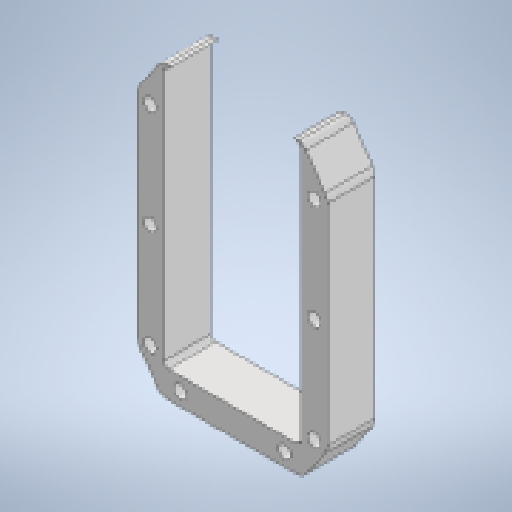
# Autodesk Inventor part: 부품70
Saved by Autodesk Inventor 2024 (Build 280153000, 153)
## iProperties
Created: 2024-09-08
Part Number: 부품70
Material: 일반
Document SubType Name: Modeling
Designer: Eungang
Density: 1 g/cm^3
Appearance: 기본값
Author: Eungang
Autodesk Inventor part; units mm, degrees
ref_plane "YZ Plane" through (0, 0, 0) normal (1, 0, 0) x (0, 1, 0)
ref_plane "XZ Plane" through (0, 0, 0) normal (0, 1, 0) x (-1, 0, 0)
ref_plane "XY Plane" through (0, 0, 0) normal (0, 0, 1) x (1, 0, 0)
sketch "스케치1" plane through (0, 0, 0) normal (0, 0, 1) x (1, 0, 0)
  arc A0 (19.8825, 4.0579) -> (19.3633, 5.7448) centre (16.8825, 4.0579) ccw projected
  line L0 (19.3633, 5.7448) -> (15.3778, 11.6059) projected
  arc A1 (15.3778, 11.6059) -> (13.7239, 12.4812) centre (13.7239, 10.4812) ccw projected
  line L1 (12.7825, 12.4812) -> (13.7239, 12.4812) projected
  arc A2 (14.2825, 10.9812) -> (12.7825, 12.4812) centre (12.7825, 10.9812) ccw projected
  line L2 (14.2825, -42.0188) -> (14.2825, 10.9812) projected
  arc A3 (13.2825, -43.0188) -> (14.2825, -42.0188) centre (13.2825, -42.0188) ccw projected
  line L3 (-13.7175, -43.0188) -> (13.2825, -43.0188) projected
  arc A4 (-14.7175, -42.0188) -> (-13.7175, -43.0188) centre (-13.7175, -42.0188) ccw projected
  line L4 (-14.7175, 10.9812) -> (-14.7175, -42.0188) projected
  arc A5 (-13.2175, 12.4812) -> (-14.7175, 10.9812) centre (-13.2175, 10.9812) ccw projected
  line L5 (-14.1589, 12.4812) -> (-13.2175, 12.4812) projected
  arc A6 (-14.1589, 12.4812) -> (-15.8128, 11.6059) centre (-14.1589, 10.4812) ccw projected
  line L6 (-15.8128, 11.6059) -> (-19.7983, 5.7448) projected
  arc A7 (-19.7983, 5.7448) -> (-20.3175, 4.0579) centre (-17.3175, 4.0579) ccw projected
  line L7 (-20.3175, 4.0579) -> (-20.3175, -40.1954) projected
  arc A8 (-20.3175, -40.1954) -> (-19.7983, -41.8823) centre (-17.3175, -40.1954) ccw projected
  line L8 (-19.7983, -41.8823) -> (-16.1104, -47.3057) projected
  arc A9 (-16.1104, -47.3057) -> (-13.6296, -48.6188) centre (-13.6296, -45.6188) ccw projected
  line L9 (-13.6296, -48.6188) -> (13.1946, -48.6188) projected
  arc A10 (13.1946, -48.6188) -> (15.6754, -47.3057) centre (13.1946, -45.6188) ccw projected
  line L10 (15.6754, -47.3057) -> (19.3633, -41.8823) projected
  arc A11 (19.3633, -41.8823) -> (19.8825, -40.1954) centre (16.8825, -40.1954) ccw projected
  line L11 (19.8825, -40.1954) -> (19.8825, 4.0579) projected
  circle A12 centre (-17.5175, 3.4812) radius 1.35 projected
  circle A13 centre (-17.5175, -18.5188) radius 1.35 projected
  circle A14 centre (-11.2175, -45.8188) radius 1.35 projected
  circle A15 centre (17.0825, 3.4812) radius 1.35 projected
  circle A16 centre (17.0825, -18.5188) radius 1.35 projected
  circle A17 centre (10.7825, -45.8188) radius 1.35 projected
  circle A18 centre (-17.5175, -40.5188) radius 1.35 projected
  circle A19 centre (17.0825, -40.5188) radius 1.35 projected
  circle A20 centre (-0.2175, -0.5188) radius 13.9 projected
  line L12 (25.5233, 26.6812) -> (19.5233, 26.6812) projected
  line L13 (19.5233, 26.6812) -> (19.5233, -57.2188) projected
  line L14 (25.5233, -57.2188) -> (19.5233, -57.2188) projected
  line L15 (25.5233, 26.6812) -> (25.5233, -57.2188) projected
  line L16 (-20.5175, 26.6812) -> (-26.5175, 26.6812) projected
  line L17 (-26.5175, 26.6812) -> (-26.5175, -57.2188) projected
  line L18 (-20.5175, -57.2188) -> (-26.5175, -57.2188) projected
  line L19 (-20.5175, 26.6812) -> (-20.5175, -57.2188) projected
  line L20 (14.2825, -40.5188) -> (19.5233, -40.5188)
  line L21 (19.5233, -40.5188) -> (19.5233, -57.2188)
  line L22 (19.5233, -57.2188) -> (14.2825, -57.2188)
  line L23 (14.2825, -57.2188) -> (14.2825, -40.5188)
  line L24 (-20.3, -40.5188) -> (-14.7175, -40.5188)
  line L25 (-14.7175, -40.5188) -> (-14.7175, -57.2188)
  line L26 (-14.7175, -57.2188) -> (-20.3, -57.2188)
  line L27 (-20.3, -57.2188) -> (-20.3, -40.5188)
  line L28 (19.865, -40.5188) -> (14.2825, -40.5188)
  line L29 (14.2825, -40.5188) -> (14.2825, -57.2188)
  line L30 (14.2825, -57.2188) -> (19.865, -57.2188)
  line L31 (19.865, -57.2188) -> (19.865, -40.5188)
  line L32 (-20.5175, -40.5188) -> (-14.7175, -40.5188)
  line L33 (-14.7175, -40.5188) -> (-14.7175, -57.2188)
  line L34 (-14.7175, -57.2188) -> (-20.5175, -57.2188)
  line L35 (-20.5175, -57.2188) -> (-20.5175, -40.5188)
  line L36 (-20.3175, 4.0579) -> (-20.5175, 4.0579)
  line L37 (19.8825, 4.0579) -> (19.5233, 4.0579)
  point P0 (0, 0)
  point P1 (14.2825, -48.4146)
  point P2 (19.5233, -41.6188)
  point P3 (-14.7175, -48.4146)
  constraints: 36 end point, 8 parallel, 6 perpendicular, 6 point on line, 4 horizontal, 2 point on circle
extrude "돌출1" add sketch "스케치1" along normal blind 12 contours L37 L13 A0 | L11 A11 L28 L13 L37 | L13 L20 A19 L2 A2 L1 A1 L0 A0 | A11 L13 L28 | L13 A11 L10 A10 L23 L2 L20 A19 | L13 L22 L23 A10 L10 A11 | A10 L9 A9 L25 A4 L3 A3 L23 | L25 L26 L27 A8 L8 A9 | A9 L8 A8 L24 A18 L4 L25 | L24 A18 A8 L7 A7 L6 A6 L5 A5 L4
sketch "스케치2" plane through (-20.3175, -40.1954, 0) normal (-1, 0, 0) x (0, 0, 1)
  line L0 (6, 66.8766) -> (6, -17.0234) projected
  line L1 (0, 0) -> (12, 0) projected
  line L2 (0, 44.2533) -> (12, 44.2533) projected
  line L3 (6, 0) -> (12, 0)
  line L4 (12, 0) -> (12, 44.2533)
  line L5 (12, 44.2533) -> (6, 44.2533)
  line L6 (6, 44.2533) -> (6, 0)
  point P0 (0, 40.1954)
  point P1 (12, 0)
  point P2 (6, 44.2533)
  point P3 (6, 0)
  constraints: 8 end point, 2 parallel, 1 horizontal, 1 midpoint, 1 perpendicular
extrude "돌출2" add sketch "스케치2" along normal blind 6
sketch "스케치3" plane through (19.8825, -40.1954, 0) normal (1, 0, 0) x (0, 0, -1)
  line L0 (0, 44.2533) -> (-12, 44.2533) projected
  line L1 (0, -1.6734) -> (0, 1.0266) projected
  line L2 (-12, 44.2533) -> (0, 44.2533)
  line L3 (0, 44.2533) -> (0, 0)
  line L4 (0, 0) -> (-12, 0)
  line L5 (-12, 0) -> (-12, 44.2533)
  point P0 (0, 40.1954)
  constraints: 8 end point, 2 parallel, 1 horizontal, 1 perpendicular, 1 point on line
extrude "돌출3" add sketch "스케치3" along normal blind 6
thicken "두껍게 하기2" operation cut thickness 0.2 both sides no extend neighbours no toward (0, 0, 1) faces at (-24.3175, -10.6932, 6)
thicken "두껍게 하기3" operation cut thickness 0.2 both sides no extend neighbours no toward (0, 0, 1) faces at (23.3992, -18.2188, 0)
sketch "스케치4" plane through (0, 0, 12) normal (0, 0, 1) x (1, 0, 0)
  line L0 (-15.8128, 11.6059) -> (-19.7983, 5.7448) projected
  arc A0 (-19.7983, 5.7448) -> (-20.3175, 4.0579) centre (-17.3175, 4.0579) ccw projected
  line L1 (-20.3175, 4.0579) -> (-26.3175, 4.0579) projected
  line L2 (-26.3175, -40.1954) -> (-26.3175, 4.0579) projected
  line L3 (-20.3175, -40.1954) -> (-26.3175, -40.1954) projected
  arc A1 (-20.3175, -40.1954) -> (-20.3, -40.5188) centre (-17.3175, -40.1954) ccw projected
  line L4 (-20.3, -40.5188) -> (-20.3, -57.2188) projected
  line L5 (-20.3, -57.2188) -> (-14.7175, -57.2188) projected
  line L6 (-14.7175, -57.2188) -> (-14.7175, -48.4146) projected
  arc A2 (-14.7175, -48.4146) -> (-13.6296, -48.6188) centre (-13.6296, -45.6188) ccw projected
  line L7 (-13.6296, -48.6188) -> (13.1946, -48.6188) projected
  arc A3 (13.1946, -48.6188) -> (14.2825, -48.4146) centre (13.1946, -45.6188) ccw projected
  line L8 (14.2825, -48.4146) -> (14.2825, -57.2188) projected
  line L9 (14.2825, -57.2188) -> (19.5233, -57.2188) projected
  line L10 (19.5233, -57.2188) -> (19.5233, -41.6188) projected
  arc A4 (19.5233, -41.6188) -> (19.8825, -40.1954) centre (16.8825, -40.1954) ccw projected
  line L11 (19.8825, -40.1954) -> (25.8825, -40.1954) projected
  line L12 (25.8825, 4.0579) -> (25.8825, -40.1954) projected
  line L13 (19.8825, 4.0579) -> (25.8825, 4.0579) projected
  arc A5 (19.8825, 4.0579) -> (19.3633, 5.7448) centre (16.8825, 4.0579) ccw projected
  line L14 (19.3633, 5.7448) -> (15.3778, 11.6059) projected
  arc A6 (15.3778, 11.6059) -> (13.7239, 12.4812) centre (13.7239, 10.4812) ccw projected
  line L15 (13.7239, 12.4812) -> (12.7825, 12.4812) projected
  arc A7 (14.2825, 10.9812) -> (12.7825, 12.4812) centre (12.7825, 10.9812) ccw projected
  line L16 (14.2825, 10.9812) -> (14.2825, -42.0188) projected
  arc A8 (13.2825, -43.0188) -> (14.2825, -42.0188) centre (13.2825, -42.0188) ccw projected
  line L17 (13.2825, -43.0188) -> (-13.7175, -43.0188) projected
  arc A9 (-14.7175, -42.0188) -> (-13.7175, -43.0188) centre (-13.7175, -42.0188) ccw projected
  line L18 (-14.7175, -42.0188) -> (-14.7175, 10.9812) projected
  arc A10 (-13.2175, 12.4812) -> (-14.7175, 10.9812) centre (-13.2175, 10.9812) ccw projected
  line L19 (-13.2175, 12.4812) -> (-14.1589, 12.4812) projected
  arc A11 (-14.1589, 12.4812) -> (-15.8128, 11.6059) centre (-14.1589, 10.4812) ccw projected
  circle A12 centre (17.0825, -40.5188) radius 1.35 projected
  circle A13 centre (-17.5175, -40.5188) radius 1.35 projected
  circle A14 centre (10.7825, -45.8188) radius 1.35 projected
  circle A15 centre (17.0825, -18.5188) radius 1.35 projected
  circle A16 centre (17.0825, 3.4812) radius 1.35 projected
  circle A17 centre (-11.2175, -45.8188) radius 1.35 projected
  circle A18 centre (-17.5175, -18.5188) radius 1.35 projected
  circle A19 centre (-17.5175, 3.4812) radius 1.35 projected
  line L20 (19.3633, -40.1954) -> (25.8825, -40.1954)
  line L21 (25.8825, -40.1954) -> (25.8825, -57.2188)
  line L22 (25.8825, -57.2188) -> (19.3633, -57.2188)
  line L23 (19.3633, -57.2188) -> (19.3633, -40.1954)
  line L24 (-26.3175, -40.1954) -> (-20.3175, -40.1954) projected
  line L25 (-20.3175, -40.1954) -> (-26.3175, -40.1954)
  line L26 (-26.3175, -40.1954) -> (-26.3175, -57.2188)
  line L27 (-26.3175, -57.2188) -> (-20.3175, -57.2188)
  line L28 (-20.3175, -57.2188) -> (-20.3175, -40.1954)
  line L29 (25.8825, 4.0579) -> (12.7825, 4.0579)
  line L30 (12.7825, 4.0579) -> (12.7825, 12.4812)
  line L31 (12.7825, 12.4812) -> (25.8825, 12.4812)
  line L32 (25.8825, 12.4812) -> (25.8825, 4.0579)
  line L33 (-26.3175, 4.0579) -> (-13.2175, 4.0579)
  line L34 (-13.2175, 4.0579) -> (-13.2175, 12.4812)
  line L35 (-13.2175, 12.4812) -> (-26.3175, 12.4812)
  line L36 (-26.3175, 12.4812) -> (-26.3175, 4.0579)
  line L37 (14.2825, 4.0579) -> (12.7825, 4.0579)
  line L38 (12.7825, 4.0579) -> (12.7825, 12.4812)
  line L39 (12.7825, 12.4812) -> (14.2825, 12.4812)
  line L40 (14.2825, 12.4812) -> (14.2825, 4.0579)
  line L41 (-13.2175, 12.4812) -> (-14.7175, 12.4812)
  line L42 (-14.7175, 12.4812) -> (-14.7175, 4.0579)
  line L43 (-14.7175, 4.0579) -> (-13.2175, 4.0579)
  line L44 (-13.2175, 4.0579) -> (-13.2175, 12.4812)
  point P0 (0, 0)
  point P1 (14.2825, 12.4017)
  point P2 (19.8825, -40.1954)
  point P3 (-14.7175, 12.4017)
  constraints: 48 end point, 12 parallel, 6 horizontal, 6 perpendicular, 5 point on line
extrude "돌출4" add sketch "스케치4" against normal blind 12 contours L0 A0 L1 L36 L35 L42 A11 | L3 L28 L27 L26 | L40 L31 L32 L13 A5 L14 A6 | L21 L22 L10 A4 L11 | L23 L20 A4 L10 L9
